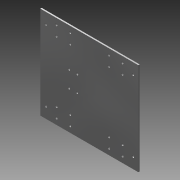
# Autodesk Inventor part: Base Plate
Saved by Autodesk Inventor 2015 (Build 190159000, 159)
## iProperties
Created: 2015-02-23
Part Number: Base Plate
Material: Aluminum 6061
Document SubType Name: Modeling
Designer: Andrew
Density: 2.7 g/cm^3
Appearance: Aluminum - Flat
Width: 180.000 mm
Author: Andrew
Autodesk Inventor part; units mm, degrees
ref_plane "YZ Plane" through (0, 0, 0) normal (1, 0, 0) x (0, 1, 0)
ref_plane "XZ Plane" through (0, 0, 0) normal (0, 1, 0) x (-1, 0, 0)
ref_plane "XY Plane" through (0, 0, 0) normal (0, 0, 1) x (1, 0, 0)
sketch "Sketch1" plane through (0, 0, 0) normal (0, 1, 0) x (-1, 0, 0)
  line L0 (90, 85) -> (-90, 85)
  line L1 (-90, 85) -> (-90, -85)
  line L2 (-90, -85) -> (90, -85)
  line L3 (90, -85) -> (90, 85)
  line L4 (0, -119) -> (0, 119) projected
  line L5 (-126, 0) -> (126, 0) projected
  point P0 (0, 0)
  dimension "Length" = 170
  dimension "Width" = 180
  constraints: 8 end point, 2 parallel, 1 horizontal, 1 perpendicular, 2 other
  measures "Length" distance of L2.end L0.start
  measures "Width" distance of L1.end L2.end
extrude "Extrusion1" add sketch "Sketch1" along normal blind 2.5
sketch "Sketch2" plane through (0, 2.5, 0) normal (0, 1, 0) x (1, 0, 0)
  circle A0 centre (-60.5, -74) radius 2.0625
  circle A1 centre (-60.5, -56) radius 2.0625
  circle A2 centre (-35.5, -74) radius 2.0625
  circle A3 centre (-35.5, -56) radius 2.0625
  line L0 (-60.5, -74) -> (-60.5, -56) construction
  line L1 (-60.5, -56) -> (-35.5, -56) construction
  line L2 (-35.5, -56) -> (-35.5, -74) construction
  line L3 (-35.5, -74) -> (-60.5, -74) construction
  line L4 (-90, 85) -> (-90, -85) construction
  line L5 (-90, -85) -> (90, -85) construction
  circle A4 centre (-80, -65) radius 2.0625
  point P0 (0, 0)
  dimension "d4" = 4.125
  dimension "d5" = 18
  dimension "d6" = 25
  dimension "d7" = 29.5
  dimension "d8" = 11
  dimension "d9" = 4.125
  dimension "d10" = 10
  dimension "d11" = 20
  constraints: 8 end point, 5 centre point, 3 equal radius, 2 perpendicular, 1 parallel, 1 vertical
  measures "d4" diameter of A0
  measures "d5" distance of L0.start L0.end
  measures "d6" distance of L2.end L0.start
  measures "d7" distance between parallel lines of L4 L0
  measures "d8" distance between parallel lines of L5 L3
  measures "d9" diameter of A4
  measures "d10" distance from line of L4 A4.centre
  measures "d11" distance from line of L5 A4.centre
extrude "Extrusion2" cut sketch "Sketch2" against normal up to next
mirror "Mirror1" about plane through (0, 0, 0) normal (0, 0, 1) of "Extrusion2"
mirror "Mirror2" about plane through (0, 0, 0) normal (1, 0, 0) of "Extrusion2", "Mirror1"
sketch "Sketch3" plane through (0, 2.5, 0) normal (0, 1, 0) x (1, 0, 0)
  circle A0 centre (-37.5, -15) radius 2.0625
  circle A1 centre (-37.5, 15) radius 2.0625
  circle A2 centre (-22.5, -15) radius 2.0625
  circle A3 centre (-22.5, 15) radius 2.0625
  line L0 (-22.5, 15) -> (-37.5, 15) construction
  line L1 (-37.5, 15) -> (-37.5, -15) construction
  line L2 (-37.5, -15) -> (-22.5, -15) construction
  line L3 (-22.5, -15) -> (-22.5, 15) construction
  line L4 (-22.5, 15) -> (-37.5, -15) construction
  line L5 (-37.5, 15) -> (-22.5, -15) construction
  line L6 (-90, 85) -> (-90, -85) construction
  line L7 (144.445, 0) -> (-144.445, 0) construction
  point P0 (0, 0)
  point P1 (-30, 0)
  point P2 (-30, 0)
  dimension "d14" = 30
  dimension "d15" = 4.125
  dimension "d16" = 15
  dimension "d17" = 60
  constraints: 14 end point, 4 centre point, 3 coincident, 3 equal radius, 3 midpoint, 2 horizontal, 2 parallel, 1 perpendicular, 1 point on line, 2 other
  measures "d14" distance between parallel lines of L0 L2
  measures "d15" diameter of A1
  measures "d16" distance between parallel lines of L3 L1
  measures "d17" distance from line of L6 point (-30, 0)
extrude "Extrusion3" cut sketch "Sketch3" against normal up to next
body "Solid1"
